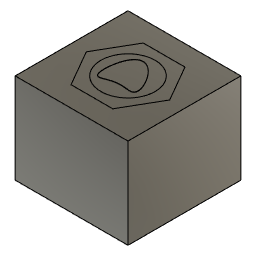
Multipart Demo v3 (Autodesk Fusion 360 design; units mm, degrees)
Autodesk Fusion 360 part; units mm, degrees
sketch "Sketch1" plane through (0, 0, 0) normal (0, 0, 1) x (1, 0, 0) in component "Multipart Demo"
  line L0 (0, 0) -> (25, 0)
  line L1 (25, 0) -> (25, 25)
  line L2 (25, 25) -> (0, 25)
  line L3 (0, 25) -> (0, 0)
  line L4 (7.8812, 20.5) -> (3.2624, 12.5)
  line L5 (3.2624, 12.5) -> (7.8812, 4.5)
  line L6 (7.8812, 4.5) -> (17.1188, 4.5)
  line L7 (17.1188, 4.5) -> (21.7376, 12.5)
  line L8 (21.7376, 12.5) -> (17.1188, 20.5)
  line L9 (17.1188, 20.5) -> (7.8812, 20.5)
  circle A0 centre (12.5, 12.5) radius 6
  spline S0 degree 5 poles (8.9094, 9.3519) (9.0191, 9.2045) (9.2754, 9.0123) (9.7707, 9.0232) (10.6665, 9.4656) (12.2037, 10.0156) (14.0226, 10.0885) (15.8151, 9.6278) (16.7222, 10.0857) (16.468, 11.7824) (15.2326, 14.1604) (13.4321, 16.3126) (11.5676, 17.3295) (10.0315, 16.7793) (8.9918, 14.9633) (8.4816, 12.5578) (8.4559, 10.8091) (8.6176, 9.8966) (8.7998, 9.4993) (8.9094, 9.3519) knots 0 0 0 0 0 0 0.066667 0.133333 0.2 0.266667 0.333333 0.4 0.466667 0.533333 0.6 0.666667 0.733333 0.8 0.866667 0.933333 1 1 1 1 1 1
  line L10 (13.9946, 9.9481) -> (16.204, 9.7727)
  point P0 (12.5, 12.5)
  point P1 (15.0993, 9.8604)
  point P2 (12.0833, 16.8393)
  dimension "d1" = 8
  dimension "d2" = 12
  constraint horizontal L0
  constraint vertical L1
  constraint horizontal L2
  constraint vertical L3
  constraint coincident L0.start L3.end
  constraint coincident P0 A0.centre
  constraint midpoint P1 L10
  measures "d1" distance of P0 L9
  measures "d2" diameter of A0
extrude "Extrude1" add sketch "Sketch1" against normal blind 20 contours L0 L1 L2 L3 | L4 L5 L6 L7 L8 L9 | A0 | S0 makes body 1 in component "Multipart Demo"
extrude "Extrude2" cut sketch "Sketch1" against normal blind 0.6 contours L4 L5 L6 L7 L8 L9 | S0 bodies 1 in component "Multipart Demo"
extrude "Extrude4" add sketch "Sketch1" against normal blind 0.6 separate body contours L4 L5 L6 L7 L8 L9 makes body 2 in component "Multipart Demo"
extrude "Extrude5" add 1 faces at (11.9592, 12.8035, -0.6) along direction (0, 0, 1) blind 0.6 on bodies 1 bodies 1 in component "Multipart Demo"
extrude "Extrude6" cut 1 faces at (11.5, 14.2321, 0) along direction (0, 0, -1) blind 0.6 on bodies 1 bodies 1 in component "Multipart Demo"
extrude "Extrude7" add sketch "Sketch1" against normal blind 0.6 separate body contours A0 | S0 makes body 3 in component "Multipart Demo"
extrude "Extrude8" cut sketch "Sketch1" against normal blind 0.6 contours S0 bodies 3 in component "Multipart Demo"
extrude "Extrude9" add sketch "Sketch1" against normal blind 0.06 contours S0 bodies 3 in component "Multipart Demo"
extrude "Extrude10" add sketch "Sketch1" against normal blind 0.6 contours S0 bodies 1 in component "Multipart Demo"
component "Multipart Demo" placed x (1, 0, 0) y (0, 1, 0) z (0, 0, 1) at (0, 0, 0)
